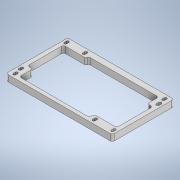
# Autodesk Inventor part: psu_spacer
Saved by Autodesk Inventor 2022 (Build 260153000, 153)
## iProperties
Created: 2021-08-12
Part Number: psu_spacer
Material: Generic
Document SubType Name: Modeling
Designer: gisen
Density: 1 g/cm^3
Appearance: Default
Author: gisen
Autodesk Inventor part; units mm, degrees
ref_plane "YZ Plane" through (0, 0, 0) normal (1, 0, 0) x (0, 1, 0)
ref_plane "XZ Plane" through (0, 0, 0) normal (0, 1, 0) x (-1, 0, 0)
ref_plane "XY Plane" through (0, 0, 0) normal (0, 0, 1) x (1, 0, 0)
sketch "Sketch1" plane through (0, 0, 0) normal (0, 1, 0) x (-1, 0, 0)
  arc A0 (-69, -145.9) -> (-66, -148.9) centre (-66, -145.9) ccw
  line L0 (-64.5, -148.9) -> (-66, -148.9)
  arc A1 (-68, -155.4) -> (-72, -155.4) centre (-70, -155.4) ccw
  line L1 (-68, -155.4) -> (-68, -158.4)
  line L2 (-72, -158.4) -> (-72, -155.4)
  arc A2 (-72, -158.4) -> (-68, -158.4) centre (-70, -158.4) ccw
  line L3 (-61.5, -162) -> (-61.5, -151.9)
  arc A3 (-66.25, -165.2) -> (-69.75, -165.2) centre (-68, -165.2) ccw
  line L4 (-66.25, -165.2) -> (-66.25, -168.2)
  line L5 (-69.75, -168.2) -> (-69.75, -165.2)
  arc A4 (-69.75, -168.2) -> (-66.25, -168.2) centre (-68, -168.2) ccw
  arc A5 (-61.5, -151.9) -> (-64.5, -148.9) centre (-64.5, -151.9) ccw
  arc A6 (61.5, -94.6) -> (58.5, -91.6) centre (58.5, -94.6) ccw
  line L6 (61.5, -94.6) -> (61.5, -107.7)
  line L7 (66.25, -94.4) -> (66.25, -91.4)
  arc A7 (69.75, -91.4) -> (66.25, -91.4) centre (68, -91.4) ccw
  line L8 (69.75, -91.4) -> (69.75, -94.4)
  arc A8 (66.25, -94.4) -> (69.75, -94.4) centre (68, -94.4) ccw
  arc A9 (71.75, -101.2) -> (68.25, -101.2) centre (70, -101.2) ccw
  line L9 (71.75, -101.2) -> (71.75, -104.2)
  arc A10 (68.25, -104.2) -> (71.75, -104.2) centre (70, -104.2) ccw
  arc A11 (61.5, -107.7) -> (64.5, -110.7) centre (64.5, -107.7) ccw
  line L10 (64.5, -110.7) -> (66, -110.7)
  arc A12 (69, -113.7) -> (66, -110.7) centre (66, -113.7) ccw
  line L11 (69, -113.7) -> (69, -158.4)
  line L12 (68.25, -104.2) -> (68.25, -101.2)
  arc A13 (66, -161.4) -> (69, -158.4) centre (66, -158.4) ccw
  arc A14 (71.75, -165.2) -> (68.25, -165.2) centre (70, -165.2) ccw
  line L13 (71.75, -165.2) -> (71.75, -168.2)
  arc A15 (68.25, -168.2) -> (71.75, -168.2) centre (70, -168.2) ccw
  line L14 (68.25, -168.2) -> (68.25, -165.2)
  line L15 (66, -161.4) -> (39.9991, -161.4)
  arc A16 (45.75, -165.4) -> (42.25, -165.4) centre (44, -165.4) ccw
  arc A17 (39.9991, -161.4) -> (37.2495, -163.2) centre (39.9991, -164.4) ccw
  line L16 (45.75, -165.4) -> (45.75, -168.4)
  arc A18 (34.5, -165) -> (37.2495, -163.2) centre (34.5, -162) ccw
  line L17 (42.25, -168.4) -> (42.25, -165.4)
  arc A19 (42.25, -168.4) -> (45.75, -168.4) centre (44, -168.4) ccw
  line L18 (34.5, -165) -> (-58.5, -165)
  arc A20 (-61.5, -162) -> (-58.5, -165) centre (-58.5, -162) ccw
  line L19 (-66, -98.4) -> (-40.5, -98.4)
  arc A21 (-71.75, -94.4) -> (-68.25, -94.4) centre (-70, -94.4) ccw
  arc A22 (-68.25, -91.4) -> (-71.75, -91.4) centre (-70, -91.4) ccw
  line L20 (-71.75, -94.4) -> (-71.75, -91.4)
  line L21 (-68.25, -91.4) -> (-68.25, -94.4)
  line L22 (-69, -145.9) -> (-69, -101.4)
  arc A23 (-66, -98.4) -> (-69, -101.4) centre (-66, -101.4) ccw
  line L23 (-45.75, -94.2) -> (-45.75, -91.2)
  arc A24 (-42.25, -91.2) -> (-45.75, -91.2) centre (-44, -91.2) ccw
  line L24 (-42.25, -91.2) -> (-42.25, -94.2)
  arc A25 (-45.75, -94.2) -> (-42.25, -94.2) centre (-44, -94.2) ccw
  line L25 (-34.5, -91.6) -> (58.5, -91.6)
  arc A26 (-34.5, -91.6) -> (-37.5, -94.6) centre (-34.5, -94.6) ccw
  line L26 (-37.5, -95.4) -> (-37.5, -94.6)
  arc A27 (-40.5, -98.4) -> (-37.5, -95.4) centre (-40.5, -95.4) ccw
  line L27 (74.75, -86.45) -> (-74.75, -86.45)
  line L28 (-74.75, -86.45) -> (-74.75, -173.15)
  line L29 (-74.75, -173.15) -> (74.75, -173.15)
  line L30 (74.75, -173.15) -> (74.75, -86.45)
  point P0 (0, 0)
  dimension "d0" = 1.75
  dimension "d1" = 3
  dimension "d2" = 2
  dimension "d3" = 2
  dimension "d4" = 2.75
  dimension "d5" = 10.25
  dimension "d6" = 26
  dimension "d7" = 109.25
  dimension "d8" = 114
  dimension "d9" = 133.25
  dimension "d10" = 138
  dimension "d11" = 139.75
  dimension "d12" = 140
  dimension "d13" = 140.75
  dimension "d14" = 50.7
  dimension "d15" = 19.1
  dimension "d16" = 54.3
  dimension "d17" = 12.3
  dimension "d18" = 38.2
  dimension "d19" = 9.5
  dimension "d20" = 6.5
  dimension "d21" = 54.5
  dimension "d22" = 57.5
  dimension "d23" = 19.3
  dimension "d24" = 16.3
  dimension "d25" = 54.7
  dimension "d26" = 57.7
  dimension "d27" = 31.7509
  dimension "d28" = 19.5
  dimension "d29" = 16.5
  dimension "d30" = 54.5
  dimension "d31" = 44.7
  dimension "d32" = 137.75
  dimension "d33" = 57.5
  dimension "d34" = 16.3
  dimension "d35" = 139
  dimension "d36" = 19.3
  dimension "d37" = 139
  dimension "d38" = 47.7
  dimension "d40" = 3
  dimension "d41" = 3
  dimension "d42" = 3
  dimension "d43" = 3
  constraints: 62 end point, 56 point on circle, 46 tangent, 28 centre point, 25 equal radius, 21 parallel, 7 perpendicular, 1 horizontal
  measures "d0" radius of A9
  measures "d1" radius of A12
  measures "d2" radius of A1
  measures "d3" distance between parallel lines of L8 L9
  measures "d4" distance between parallel lines of L11 L9
  measures "d5" distance between parallel lines of L6 L9
  measures "d6" distance between parallel lines of L9 L16
  measures "d7" distance between parallel lines of L26 L9
  measures "d8" distance between parallel lines of L9 L24
  measures "d9" distance between parallel lines of L3 L9
  measures "d10" distance between parallel lines of L4 L9
  measures "d11" distance between parallel lines of L1 L9
  measures "d12" distance between parallel lines of L9 L21
  measures "d13" distance between parallel lines of L22 L9
  measures "d14" distance between parallel lines of L10 L15
  measures "d15" distance between parallel lines of L25 L10
  measures "d16" distance between parallel lines of L18 L10
  measures "d17" distance between parallel lines of L10 L19
  measures "d18" distance between parallel lines of L0 L10
  measures "d19" distance from line of L9.start L10
  measures "d20" distance from line of L9.end L10
  measures "d21" distance from line of L13.start L10
  measures "d22" distance from line of L13.end L10
  measures "d23" distance from line of L8.start L10
  measures "d24" distance from line of L8.end L10
  measures "d25" distance from line of L16.start L10
  measures "d26" distance from line of L16.end L10
  measures "d27" distance from line of L15.end L9
  measures "d28" distance from line of L24.start L10
  measures "d29" distance from line of L24.end L10
  measures "d30" distance from line of L4.start L10
  measures "d31" distance from line of L1.start L10
  measures "d32" distance from line of A4.centre L8
  measures "d33" distance from line of A4.centre L10
  measures "d34" distance from line of L21.end L10
  measures "d35" distance from line of A22.centre L11
  measures "d36" distance from line of A22.centre L10
  measures "d37" distance from line of A2.centre L11
  measures "d38" distance from line of A2.centre L10
  measures "d40" distance edge to line of A19 L29
  measures "d41" distance between parallel lines of L13 L30
  measures "d42" distance edge to line of A24 L27
  measures "d43" distance between parallel lines of L20 L28
extrude "Extrusion1" add sketch "Sketch1" along normal blind 9
fillet "Fillet1" radius 3 4 edges at (-74.75, 4.5, -86.45) (-74.75, 4.5, -173.15) (74.75, 4.5, -173.15) (74.75, 4.5, -86.45)
body "Solid1"
